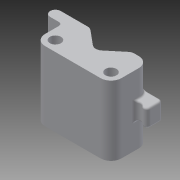
# Autodesk Inventor part: holder
Saved by Autodesk Inventor 2014 (Build 180170000, 170)
## iProperties
Created: 2018-06-15
Part Number: holder
Material: Všeobecné
Document SubType Name: Modeling
Designer: Vojta3310
Density: 1 g/cm^3
Appearance: Výchozí
Author: Vojta3310
Autodesk Inventor part; units mm, degrees
ref_plane "YZ Plane" through (0, 0, 0) normal (1, 0, 0) x (0, 1, 0)
ref_plane "XZ Plane" through (0, 0, 0) normal (0, 1, 0) x (-1, 0, 0)
ref_plane "XY Plane" through (0, 0, 0) normal (0, 0, 1) x (1, 0, 0)
sketch "Náčrt1" plane through (0, 0, 0) normal (0, 0, 1) x (1, 0, 0)
  circle A0 centre (0, 0) radius 1.6
  circle A1 centre (16, 0) radius 1.6
  arc A2 (-3, 0) -> (0, -3) centre (0, 0) ccw
  arc A3 (16, -3) -> (19, 0) centre (16, 0) ccw
  line L0 (0, -3) -> (16, -3)
  line L1 (-3, 0) -> (-3, 8)
  line L2 (-3, 8) -> (2, 8)
  line L3 (2, 8) -> (8, 3)
  line L4 (8, 3) -> (14, 8)
  line L5 (14, 8) -> (19, 8)
  line L6 (19, 8) -> (19, 0)
  dimension "d0" = 3.2
  dimension "d1" = 3.2
  dimension "d2" = 16
  dimension "d3" = 6
  dimension "d4" = 6
  dimension "d5" = 8
  dimension "d6" = 8
  dimension "d7" = 12
  dimension "d8" = 5
  constraints: 14 end point, 4 centre point, 4 point on circle, 4 tangent, 3 coincident, 3 perpendicular, 2 equal length, 1 collinear, 1 horizontal alignment
  measures "d0" diameter of A0
  measures "d1" diameter of A1
  measures "d2" distance of A1.centre A0.centre
  measures "d3" diameter of A2
  measures "d4" diameter of A3
  measures "d5" distance from line of L2 point (0, 0)
  measures "d6" distance from line of A1.centre L5
  measures "d7" distance of L4.end L2.end
  measures "d8" distance from line of L2 L3.end
extrude "Vysunutí1" add sketch "Náčrt1" along normal blind 20
fillet "Zaoblení1" radius 2 3 edges at (2, 8, 10) (14, 8, 10) (8, 3, 10)
sketch "Náčrt2" plane through (19, 0, 0) normal (1, 0, 0) x (0, 0, -1)
  line L0 (0, 8) -> (-20, 8) projected
  line L1 (-20, 0) -> (-20, 8) projected
  line L2 (-12.5, 8) -> (-7.5, 8)
  line L3 (-7.5, 8) -> (-7.5, 3)
  line L4 (-7.5, 3) -> (-12.5, 3)
  line L5 (-12.5, 3) -> (-12.5, 8)
  point P0 (0, 0)
  dimension "d13" = 20
  dimension "d14" = 5
  dimension "d15" = 7.5
  dimension "d16" = 5
  constraints: 8 end point, 2 parallel, 1 horizontal, 1 perpendicular, 1 point on line
  measures "d13" distance of point (0, 0) L1.start
  measures "d14" distance of L3.end L4.end
  measures "d15" distance between parallel lines of L5 L1
  measures "d16" distance of L4.end L2.start
extrude "Vysunutí2" add sketch "Náčrt2" along normal blind 4
sketch "Náčrt3" plane through (19, 3, 12.5) normal (0, 0, 1) x (1, 0, 0)
  line L0 (0, 0) -> (4, 0) projected
  circle A0 centre (1.25, 0) radius 1.25
  line L1 (0, -3) -> (0, 5) projected
  point P0 (-19, -3)
  dimension "d19" = 2.5
  constraints: 1 centre point, 1 point on line, 1 tangent
  measures "d19" diameter of A0
extrude "Vysunutí3" cut sketch "Náčrt3" against normal through all
fillet "Zaoblení3" radius 1 3 edges at (19, 3, 10) (21.5, 3, 10) (23, 3, 10)
fillet "Zaoblení4" radius 1 1 edges at (23, 8, 10)
fillet "Zaoblení5" radius 3 2 edges at (19, 8, 16.25) (19, 8, 3.75)
fillet "Zaoblení6" radius 0.5 1 edges at (18.1213, 7.1213, 12.5)
fillet "Zaoblení7" radius 0.5 6 edges at (16.8855, 8, 12.666) (22.7071, 7.7071, 12.5) (23, 5.707, 12.5) (22.3333, 3.4712, 12.5) (20.4044, 4.2404, 12.5) (18.4014, 8, 12.5)
fillet "Zaoblení8" radius 0.5 1 edges at (18.1213, 7.1213, 7.5)
fillet "Zaoblení9" radius 0.5 6 edges at (22.7071, 7.7071, 7.5) (23, 5.707, 7.5) (22.3333, 3.4712, 7.5) (20.4044, 4.2404, 7.5) (16.8855, 8, 7.334) (18.4014, 8, 7.5)
sketch "Náčrt4" plane through (-3, 0, 0) normal (-1, 0, 0) x (0, 0, 1)
  line L0 (20, 8) -> (20, 0) projected
  line L1 (0, 8) -> (20, 8)
  line L2 (20, 8) -> (20, 5)
  line L3 (20, 5) -> (0, 5)
  line L4 (0, 5) -> (0, 8)
  dimension "d29" = 3
  constraints: 8 end point, 2 parallel, 1 horizontal, 1 perpendicular, 1 point on line
  measures "d29" distance of L3.end L1.start
extrude "Vysunutí4" add sketch "Náčrt4" along normal blind 5
fillet "Zaoblení11" radius 1.5 2 edges at (-8, 8, 10) (-8, 5, 10)
fillet "Zaoblení12" radius 1 1 edges at (-3, 5, 10)
sketch "Náčrt5" plane through (-6.5, 5, 0) normal (0, -1, 0) x (1, 0, 0)
  line L0 (2.5, 20) -> (0, 20) projected
  line L1 (0, 0) -> (0, 20) projected
  point P0 (2.5, 0)
  point P1 (6.5, 0)
  point P2 (1.25, 13)
  point P3 (1.25, 7)
  dimension "d35" = 2.5
  dimension "d36" = 1.25
  dimension "d37" = 6
  dimension "d38" = 20
  dimension "d39" = 7
  constraints: 1 vertical alignment
  measures "d35" distance of point (2.5, 0) L1.start
  measures "d36" distance from line of L1 point (1.25, 7)
  measures "d37" distance of point (1.25, 7) point (1.25, 13)
  measures "d38" distance of L1.start L0.end
  measures "d39" distance from line of L0 point (1.25, 13)
hole "Díra1" at (-5.25, 5, 13) at (-5.25, 5, 7) direction (0, 1, 0) diameter 2 end through all
equation "\"d6\" = d5"
equation "\"d15\" = -0.5 * d14 + 0.5 * d13"
equation "\"d36\" = 0.5 * d35"
equation "\"d39\" = -0.5 * d37 + 0.5 * d38"
